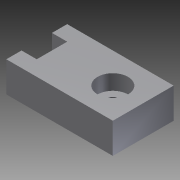
# Autodesk Inventor part: lesson1
Saved by Autodesk Inventor 2011 SP1 (Build 150282100, 282)
## iProperties
Created: 2011-10-07
Part Number: lesson1
Material: Default
Document SubType Name: Sheet Metal
Designer: Kevin
Density: 1 g/cm^3
Sheet Metal Rule: Default_mm
Author: Kevin
Autodesk Inventor part; units mm, degrees
ref_plane "YZ Plane" through (0, 0, 0) normal (1, 0, 0) x (0, 1, 0)
ref_plane "XZ Plane" through (0, 0, 0) normal (0, 1, 0) x (-1, 0, 0)
ref_plane "XY Plane" through (0, 0, 0) normal (0, 0, 1) x (1, 0, 0)
sketch "Sketch1" plane through (0, 0, 0) normal (0, 0, 1) x (1, 0, 0)
  line L0 (-25, 10) -> (10, 10)
  line L1 (10, 10) -> (10, -10)
  line L2 (10, -10) -> (-25, -10)
  line L3 (-25, 5) -> (-20, 5)
  line L4 (-20, 5) -> (-20, -5)
  line L5 (-20, -5) -> (-25, -5)
  line L6 (-25, -10) -> (-25, -5)
  line L7 (-25, 5) -> (-25, 10)
  circle A0 centre (0, 0) radius 2.5
  point P0 (10, 0)
  dimension "d0" = 5
  dimension "d1" = 10
  dimension "d2" = 5
  dimension "d3" = 5
  dimension "d4" = 5
  dimension "d5" = 35
  dimension "d7" = 10
  dimension "d8" = 5
  constraints: 16 end point, 6 perpendicular, 3 parallel, 1 centre point, 1 coincident, 1 horizontal, 1 horizontal alignment, 1 midpoint
  measures "d0" distance of L3.start L0.start
  measures "d1" distance of L3.end L4.end
  measures "d2" distance of L2.end L5.end
  measures "d3" distance between parallel lines of L4 L7
  measures "d4" distance between parallel lines of L4 L6
  measures "d5" distance between parallel lines of L1 L6
  measures "d7" distance of point (10, 0) A0.centre
  measures "d8" diameter of A0
extrude "Extrusion1" add sketch "Sketch1" along normal blind 10
sketch "Sketch2" plane through (0, 0, 10) normal (0, 0, 1) x (1, 0, 0)
  circle A0 centre (0, 0) radius 2.5 projected
  circle A1 centre (0, 0) radius 5
  dimension "d11" = 10
  constraints: 1 centre point, 1 coincident
  measures "d11" diameter of A1
extrude "Extrusion2" cut sketch "Sketch2" against normal blind 5
equation "\"BendRadius\" = Thickness"
equation "\"BendReliefWidth\" = Thickness"
equation "\"BendReliefDepth\" = 0.5 * Thickness"
equation "\"CornerReliefSize\" = 4 * Thickness"
equation "\"MinimumRemnant\" = 2 * Thickness"
equation "\"TransitionRadius\" = BendRadius"
equation "\"JacobiRadiusSize\" = BendRadius"
equation "\"GapSize\" = Thickness"
equation "\"Thickness\" = 0.5"
body "Solid1"
